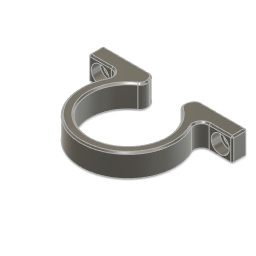
_GPS holder.9b4c6a14-adf5-428e-8618-3bced4a97906 (Autodesk Fusion 360 design; units mm, degrees)
Autodesk Fusion 360 part; units mm, degrees
note: some values were not read from the file. Set by a fixed rule: which face or edge a step refers to.
sketch "Sketch1" plane through (0, 0, 0) normal (0, 1, 0) x (1, 0, 0)
  circle A0 centre (0, 0) radius 12.75
  circle A1 centre (0, 0) radius 15.75
  line L0 (0, 0) -> (0, 15.75)
  line L1 (24, 10.75) -> (24, 15.75)
  line L2 (24, 15.75) -> (0, 15.75)
  line L3 (11.5109, 10.75) -> (24, 10.75)
  line L4 (0, 12.75) -> (0, 15.75)
  line L5 (5.5761, 11.466) -> (6.606, 14.2976)
  line L6 (-5.5761, 11.466) -> (-6.606, 14.2976)
  line L7 (6.606, 14.2976) -> (7.1343, 15.75)
  dimension "d1" = 25.5
  dimension "d2" = 3
  dimension "d3" = 24
  dimension "d4" = 5
  dimension "d5" = 12.4891
  constraint coincident A0.centre A1.centre
  constraint concentric A0 A1
  constraint coincident A1 L0.end
  constraint vertical L0
  constraint perpendicular L1 L2
  constraint coincident A1 L3.start
  constraint horizontal L2
  constraint horizontal L3
  constraint coincident L0 L4.start
  constraint coincident A0 L4.start
  constraint coincident A0 L5.start
  constraint coincident A1 L5.end
  constraint symmetric L0 L5.start L6.start
  constraint symmetric L0 L5.end L6.end
  constraint coincident L2 L7.end
  constraint parallel L5 L7
  measures "d1" diameter of A0
  measures "d2" distance of A0 A1
  measures "d3" distance of L0.end L1.end
  measures "d4" distance of L1.start L1.end
  measures "d5" distance of L1.start L3.start
extrude "Extrude1" add sketch "Sketch1" along normal blind 8 contours A0 A1 L5 L6 makes body 1
extrude "Extrude2" add sketch "Sketch1" along normal blind 8 separate body contours A1 L1 L2 L3 L7 makes body 2
sketch "Sketch2" plane through (0, 0, -10.75) normal (0, 0, 1) x (1, 0, 0)
  line L0 (11.5109, 0) -> (24, 0)
  line L1 (24, 0) -> (24, 8)
  line L2 (24, 8) -> (11.5109, 8)
  line L3 (11.5109, 8) -> (11.5109, 0)
  circle A0 centre (20, 4) radius 3
  circle A1 centre (20, 4) radius 1.9
  line L4 (0, 0) -> (0, 7)
  line L5 (24, 4) -> (20, 4)
  dimension "d10" = 20
  dimension "d11" = 3.8
  dimension "d12" = 6
  constraint concentric A0 A1
  constraint coincident L4.start origin
  constraint vertical L4
  constraint midpoint L1 L5.start
  constraint coincident A0.centre A1.centre
  constraint horizontal L5
  measures "d10" distance of A0.centre L4
  measures "d11" diameter of A1
  measures "d12" diameter of A0
extrude "Extrude3" cut sketch "Sketch2" against normal blind 9 contours A1 bodies 2
extrude "Extrude4" cut sketch "Sketch2" against normal blind 3 contours A0 bodies 2
mirror "Mirror1" about plane through (0, 0, 0) normal (1, 0, 0) of bodies 2 makes body 3
combine "Combine1" operation add target body 3 tool bodies 1 2
fillet "Fillet1" radius 2.5 6 edges at (11.5109, 4, -10.75) (-11.5109, 4, -10.75) (-5.5761, 4, -11.466) (5.5761, 4, -11.466) (7.1343, 4, -15.75) (-7.1343, 4, -15.75) on bodies 3
chamfer "Chamfer1" distance 0.5 angle 45 28 edges at (0, 8, 15.75) (14.1486, 8, -9.5586) (20.1394, 8, -10.75) (-20.1394, 8, -10.75) (-14.1486, 8, -9.5586) (0, 8, 12.75) (-6.2564, 8, -11.8057) (-6.4118, 8, -13.7636) (-7.451, 8, -15.2977) (-16.4426, 8, -15.75) (16.4426, 8, -15.75) (7.451, 8, -15.2977) (6.4118, 8, -13.7636) (6.2564, 8, -11.8057) (0, 0, 15.75) (14.1486, 0, -9.5586) (20.1394, 0, -10.75) (-20.1394, 0, -10.75) (-14.1486, 0, -9.5586) (0, 0, 12.75) (6.2564, 0, -11.8057) (6.4118, 0, -13.7636) (7.451, 0, -15.2977) (16.4426, 0, -15.75) (-16.4426, 0, -15.75) (-7.451, 0, -15.2977) (-6.4118, 0, -13.7636) (-6.2564, 0, -11.8057) 2 faces at (-24, 5.3333, -12.4167) (24, 5.3333, -12.4167) on bodies 3
equation "d15 = -5.00 mm + 2 mm"
